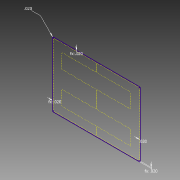
# Autodesk Inventor part: twine
Saved by Autodesk Inventor 2015 (Build 190159000, 159)
## iProperties
Created: 2014-10-08
Part Number: twine
Material: Polypropylene
Document SubType Name: Modeling
Designer: Adam
Density: 0.899 g/cm^3
Appearance: Fine Textured - Black
Author: Adam
Autodesk Inventor part; units mm, degrees
ref_plane "YZ Plane" through (0, 0, 0) normal (1, 0, 0) x (0, 1, 0)
ref_plane "XZ Plane" through (0, 0, 0) normal (0, 1, 0) x (-1, 0, 0)
ref_plane "XY Plane" through (0, 0, 0) normal (0, 0, 1) x (1, 0, 0)
sketch "Sketch1" plane through (0, 0, 0) normal (0, 0, 1) x (1, 0, 0)
  line L0 (23.8, -34.93) -> (0, -34.93) construction
  line L1 (23.8, -30.365) -> (23.8, -34.93) construction
  line L2 (4.75, -30.365) -> (23.8, -30.365) construction
  line L3 (4.75, -22.23) -> (4.75, -30.365) construction
  line L4 (23.8, -22.23) -> (4.75, -22.23) construction
  line L5 (23.8, -12.7) -> (23.8, -22.23) construction
  line L6 (4.75, -12.7) -> (23.8, -12.7) construction
  line L7 (4.75, -4.565) -> (4.75, -12.7) construction
  line L8 (23.8, -4.565) -> (4.75, -4.565) construction
  line L9 (23.8, 0) -> (23.8, -4.565) construction
  line L10 (0, 0) -> (23.8, 0) construction
  line L11 (0, -34.93) -> (0, 0) construction
  line L12 (23.8, 0) -> (47.6, 0) construction
  line L13 (23.8, -4.565) -> (23.8, 0) construction
  line L14 (42.85, -4.565) -> (23.8, -4.565) construction
  line L15 (42.85, -12.7) -> (42.85, -4.565) construction
  line L16 (23.8, -12.7) -> (42.85, -12.7) construction
  line L17 (23.8, -22.23) -> (23.8, -12.7) construction
  line L18 (42.85, -22.23) -> (23.8, -22.23) construction
  line L19 (42.85, -30.365) -> (42.85, -22.23) construction
  line L20 (23.8, -30.365) -> (42.85, -30.365) construction
  line L21 (23.8, -34.93) -> (23.8, -30.365) construction
  line L22 (47.6, -34.93) -> (23.8, -34.93) construction
  line L23 (47.6, 0) -> (47.6, -34.93) construction
  line L24 (0, 0.5) -> (47.6, 0.5)
  line L25 (48.1, 0) -> (48.1, -34.93)
  line L26 (47.6, -35.43) -> (0, -35.43)
  line L27 (-0.5, -34.93) -> (-0.5, 0)
  arc A0 (0, 0.5) -> (-0.5, 0) centre (0, 0) ccw
  arc A1 (-0.5, -34.93) -> (0, -35.43) centre (0, -34.93) ccw
  arc A2 (47.6, -35.43) -> (48.1, -34.93) centre (47.6, -34.93) ccw
  arc A3 (48.1, 0) -> (47.6, 0.5) centre (47.6, 0) ccw
  dimension "d0" = 0.5
  dimension "d1" = 0.5
  dimension "d2" = 0.5
  dimension "d3" = 0.5
  dimension "d4" = 0.5
  constraints: 8 end point, 8 point on circle, 8 tangent, 4 centre point, 3 equal radius, 2 parallel, 1 horizontal, 1 perpendicular
  measures "d0" distance between parallel lines of L23 L25
  measures "d1" distance between parallel lines of L22 L26
  measures "d2" distance between parallel lines of L27 L11
  measures "d3" distance between parallel lines of L10 L24
  measures "d4" radius of A0
sketch "Sketch2" plane through (0, 0, 0) normal (1, 0, 0) x (0, 1, 0)
  circle A0 centre (0.5, 0) radius 0.25 construction
  circle A1 centre (0.7023, 0.1469) radius 0.1469
  circle A2 centre (0.4227, 0.2378) radius 0.1469
  circle A3 centre (0.25, 0) radius 0.1469
  circle A4 centre (0.4227, -0.2378) radius 0.1469
  circle A5 centre (0.7023, -0.1469) radius 0.1469
  line L0 (0.5, 0) -> (0, 0) construction
  point P0 (0.5, 0)
  dimension "d5" = 0.5
  constraints: 9 equal radius, 6 centre point, 5 point on circle, 2 end point, 1 coincident, 1 horizontal, 1 midpoint
  measures "d5" diameter of A0
sweep "Sweep1" add profiles "Sketch2" path "Sketch1" contours A1 | A2 | A5 | A3 | A4
equation "\"d1\" = d0"
equation "\"d2\" = d0"
equation "\"d3\" = d0"
body "Solid1"
